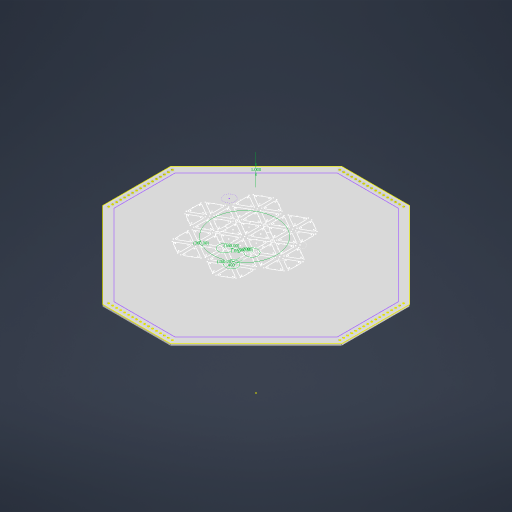
# Autodesk Inventor part: Belly Pan
Saved by Autodesk Inventor 2024.3 (Build 283343000, 343)
## iProperties
Created: 2024-11-27
Part Number: Belly Pan
Material: Generic
Document SubType Name: Modeling
Designer: kaito
Density: 1 g/cm^3
Appearance: Default
Author: kaito
Autodesk Inventor part; units mm, degrees
(part 1 of 2)
ref_plane "YZ Plane" through (0, 0, 0) normal (1, 0, 0) x (0, 1, 0)
ref_plane "XZ Plane" through (0, 0, 0) normal (0, 1, 0) x (-1, 0, 0)
ref_plane "XY Plane" through (0, 0, 0) normal (0, 0, 1) x (1, 0, 0)
sketch "Sketch1" plane through (0, 0, 0) normal (0, 1, 0) x (-1, 0, 0)
  line L0 (0, 0) -> (762, 0) construction
  line L1 (762, 0) -> (762, -762)
  line L2 (762, -762) -> (0, -762)
  line L3 (762, -273.05) -> (736.6, -273.05) construction
  line L4 (736.6, -273.05) -> (736.6, -488.95) construction
  line L5 (736.6, -488.95) -> (762, -488.95) construction
  line L6 (762, -488.95) -> (762, -273.05) construction
  line L7 (488.95, 0) -> (273.05, 0)
  line L8 (273.05, 0) -> (273.05, -25.4) construction
  line L9 (273.05, -25.4) -> (488.95, -25.4) construction
  line L10 (488.95, -25.4) -> (488.95, 0) construction
  line L11 (488.95, -762) -> (273.05, -762) construction
  line L12 (273.05, -762) -> (273.05, -736.6) construction
  line L13 (273.05, -736.6) -> (488.95, -736.6) construction
  line L14 (488.95, -736.6) -> (488.95, -762) construction
  line L15 (0, 0) -> (0, -762)
  line L16 (0, -273.05) -> (25.4, -273.05) construction
  line L17 (25.4, -273.05) -> (25.4, -488.95) construction
  line L18 (25.4, -488.95) -> (0, -488.95) construction
  line L19 (0, -488.95) -> (0, -273.05) construction
  line L20 (273.05, 0) -> (0, -273.05)
  line L21 (488.95, 0) -> (762, -273.05)
  line L22 (762, -488.95) -> (488.95, -762)
  line L23 (0, -488.95) -> (273.05, -762)
  circle A0 centre (482.6, -12.7) radius 2.4892
  circle A1 centre (469.9, -12.7) radius 2.4892
  circle A2 centre (457.2, -12.7) radius 2.4892
  circle A3 centre (444.5, -12.7) radius 2.4892
  circle A4 centre (431.8, -12.7) radius 2.4892
  circle A5 centre (419.1, -12.7) radius 2.4892
  circle A6 centre (406.4, -12.7) radius 2.4892
  circle A7 centre (393.7, -12.7) radius 2.4892
  circle A8 centre (381, -12.7) radius 2.4892
  circle A9 centre (368.3, -12.7) radius 2.4892
  circle A10 centre (355.6, -12.7) radius 2.4892
  circle A11 centre (342.9, -12.7) radius 2.4892
  circle A12 centre (330.2, -12.7) radius 2.4892
  circle A13 centre (317.5, -12.7) radius 2.4892
  circle A14 centre (304.8, -12.7) radius 2.4892
  circle A15 centre (292.1, -12.7) radius 2.4892
  circle A16 centre (279.4, -12.7) radius 2.4892
  circle A17 centre (749.3, -279.4) radius 2.4892
  circle A18 centre (749.3, -292.1) radius 2.4892
  circle A19 centre (749.3, -304.8) radius 2.4892
  circle A20 centre (749.3, -317.5) radius 2.4892
  circle A21 centre (749.3, -330.2) radius 2.4892
  circle A22 centre (749.3, -342.9) radius 2.4892
  circle A23 centre (749.3, -355.6) radius 2.4892
  circle A24 centre (749.3, -368.3) radius 2.4892
  circle A25 centre (749.3, -381) radius 2.4892
  circle A26 centre (749.3, -393.7) radius 2.4892
  circle A27 centre (749.3, -406.4) radius 2.4892
  circle A28 centre (749.3, -419.1) radius 2.4892
  circle A29 centre (749.3, -431.8) radius 2.4892
  circle A30 centre (749.3, -444.5) radius 2.4892
  circle A31 centre (749.3, -457.2) radius 2.4892
  circle A32 centre (749.3, -469.9) radius 2.4892
  circle A33 centre (749.3, -482.6) radius 2.4892
  circle A34 centre (482.6, -749.3) radius 2.4892
  circle A35 centre (469.9, -749.3) radius 2.4892
  circle A36 centre (457.2, -749.3) radius 2.4892
  circle A37 centre (444.5, -749.3) radius 2.4892
  circle A38 centre (431.8, -749.3) radius 2.4892
  circle A39 centre (419.1, -749.3) radius 2.4892
  circle A40 centre (406.4, -749.3) radius 2.4892
  circle A41 centre (393.7, -749.3) radius 2.4892
  circle A42 centre (381, -749.3) radius 2.4892
  circle A43 centre (368.3, -749.3) radius 2.4892
  circle A44 centre (355.6, -749.3) radius 2.4892
  circle A45 centre (342.9, -749.3) radius 2.4892
  circle A46 centre (330.2, -749.3) radius 2.4892
  circle A47 centre (317.5, -749.3) radius 2.4892
  circle A48 centre (304.8, -749.3) radius 2.4892
  circle A49 centre (292.1, -749.3) radius 2.4892
  circle A50 centre (279.4, -749.3) radius 2.4892
  circle A51 centre (12.7, -279.4) radius 2.4892
  circle A52 centre (12.7, -292.1) radius 2.4892
  circle A53 centre (12.7, -304.8) radius 2.4892
  circle A54 centre (12.7, -317.5) radius 2.4892
  circle A55 centre (12.7, -330.2) radius 2.4892
  circle A56 centre (12.7, -342.9) radius 2.4892
  circle A57 centre (12.7, -355.6) radius 2.4892
  circle A58 centre (12.7, -368.3) radius 2.4892
  circle A59 centre (12.7, -381) radius 2.4892
  circle A60 centre (12.7, -393.7) radius 2.4892
  circle A61 centre (12.7, -406.4) radius 2.4892
  circle A62 centre (12.7, -419.1) radius 2.4892
  circle A63 centre (12.7, -431.8) radius 2.4892
  circle A64 centre (12.7, -444.5) radius 2.4892
  circle A65 centre (12.7, -457.2) radius 2.4892
  circle A66 centre (12.7, -469.9) radius 2.4892
  circle A67 centre (12.7, -482.6) radius 2.4892
  point P0 (736.6, -381)
  point P1 (381, -25.4)
  point P2 (381, 0)
  point P3 (381, -736.6)
  point P4 (381, -762)
  point P5 (25.4, -381)
  point P6 (0, -381)
  point P7 (762, -381)
  point P8 (12.7, -273.05)
  point P9 (12.7, -488.95)
  point P10 (488.95, -12.7)
  point P11 (749.3, -273.05)
  point P12 (488.95, -749.3)
  point P13 (273.05, -762)
  point P14 (762, -488.95)
  point P15 (0, -381)
  dimension "d0" = 762
  dimension "d1" = 762
  dimension "d4" = 25.4
  dimension "d5" = 215.9
  dimension "d6" = 25.4
  dimension "d7" = 215.9
  dimension "d8" = 25.4
  dimension "d9" = 25.4
  dimension "d11" = 215.9
  dimension "d22" = 4.9784
  dimension "d23" = 6.35
  dimension "d26" = 12.7
  dimension "d31" = 4.9784
  dimension "d32" = 6.35
  dimension "d35" = 12.7
  dimension "d40" = 4.9784
  dimension "d41" = 6.35
  dimension "d44" = 12.7
  dimension "d51" = 215.9
  dimension "d60" = 4.9784
  dimension "d63" = 12.7
  constraints: 68 centre point, 48 end point, 14 midpoint, 9 parallel, 7 horizontal, 5 horizontal alignment, 5 perpendicular, 4 point on line, 4 vertical alignment, 3 vertical, 128 other
  measures "d0" distance of L1.end L2.end
  measures "d1" distance of L0.end L1.end
  measures "d4" distance of L5.end L4.end
  measures "d5" distance of L9.end L8.end
  measures "d6" distance of L8.end L7.end
  measures "d7" distance of L12.end L13.end
  measures "d8" distance of L11.end L12.end
  measures "d9" distance of L17.end L18.end
  measures "d11" distance of L3.end L4.end
  measures "d22" diameter of A0
  measures "d23" distance from line of L10 A0.centre
  measures "d26" distance of A0.centre A1.centre
  measures "d31" diameter of A17
  measures "d32" distance of point (749.3, -273.05) A17.centre
  measures "d35" distance of A17.centre A18.centre
  measures "d40" diameter of A34
  measures "d41" distance of A34.centre point (488.95, -749.3)
  measures "d44" distance of A34.centre A35.centre
  measures "d51" distance of L16.end L17.end
  measures "d60" diameter of A51
  measures "d63" distance of A51.centre A52.centre
extrude "Extrusion1" add sketch "Sketch1" along normal blind 6.35 contours L1 L22 L2 L23 L15 L20 L7 L21
sketch "Sketch3" plane through (0, 6.35, 0) normal (0, 1, 0) x (1, 0, 0)
  line L0 (-762, 488.95) -> (-762, 273.05) projected
  line L1 (-762, 273.05) -> (-488.95, 0) projected
  line L2 (-273.05, 0) -> (0, 273.05) projected
  line L3 (0, 273.05) -> (0, 488.95) projected
  line L4 (0, 488.95) -> (-273.05, 762) projected
  line L5 (-273.05, 762) -> (-488.95, 762) projected
  line L6 (-488.95, 762) -> (-762, 488.95) projected
  line L7 (-762, 488.95) -> (-762, 273.05) projected
  line L8 (-762, 273.05) -> (-488.95, 0) projected
  line L9 (-488.95, 0) -> (-273.05, 0) projected
  circle A0 centre (-12.7, 482.6) radius 2.4892 projected
  circle A1 centre (-12.7, 457.2) radius 2.4892 projected
  circle A2 centre (-12.7, 431.8) radius 2.4892 projected
  circle A3 centre (-12.7, 406.4) radius 2.4892 projected
  circle A4 centre (-12.7, 381) radius 2.4892 projected
  circle A5 centre (-12.7, 355.6) radius 2.4892 projected
  circle A6 centre (-12.7, 330.2) radius 2.4892 projected
  circle A7 centre (-12.7, 304.8) radius 2.4892 projected
  circle A8 centre (-12.7, 279.4) radius 2.4892 projected
  circle A9 centre (-292.1, 749.3) radius 2.4892 projected
  circle A10 centre (-317.5, 749.3) radius 2.4892 projected
  circle A11 centre (-342.9, 749.3) radius 2.4892 projected
  circle A12 centre (-368.3, 749.3) radius 2.4892 projected
  circle A13 centre (-393.7, 749.3) radius 2.4892 projected
  circle A14 centre (-419.1, 749.3) radius 2.4892 projected
  circle A15 centre (-444.5, 749.3) radius 2.4892 projected
  circle A16 centre (-469.9, 749.3) radius 2.4892 projected
  circle A17 centre (-749.3, 482.6) radius 2.4892 projected
  circle A18 centre (-749.3, 457.2) radius 2.4892 projected
  circle A19 centre (-749.3, 431.8) radius 2.4892 projected
  circle A20 centre (-749.3, 406.4) radius 2.4892 projected
  circle A21 centre (-749.3, 381) radius 2.4892 projected
  circle A22 centre (-749.3, 355.6) radius 2.4892 projected
  circle A23 centre (-749.3, 330.2) radius 2.4892 projected
  circle A24 centre (-749.3, 304.8) radius 2.4892 projected
  circle A25 centre (-749.3, 279.4) radius 2.4892 projected
  circle A26 centre (-292.1, 12.7) radius 2.4892 projected
  circle A27 centre (-317.5, 12.7) radius 2.4892 projected
  circle A28 centre (-342.9, 12.7) radius 2.4892 projected
  circle A29 centre (-368.3, 12.7) radius 2.4892 projected
  circle A30 centre (-393.7, 12.7) radius 2.4892 projected
  circle A31 centre (-482.6, 12.7) radius 2.4892 projected
  circle A32 centre (-469.9, 12.7) radius 2.4892 projected
  circle A33 centre (-457.2, 12.7) radius 2.4892 projected
  circle A34 centre (-444.5, 12.7) radius 2.4892 projected
  circle A35 centre (-431.8, 12.7) radius 2.4892 projected
  circle A36 centre (-419.1, 12.7) radius 2.4892 projected
  circle A37 centre (-406.4, 12.7) radius 2.4892 projected
  circle A38 centre (-381, 12.7) radius 2.4892 projected
  circle A39 centre (-355.6, 12.7) radius 2.4892 projected
  circle A40 centre (-330.2, 12.7) radius 2.4892 projected
  circle A41 centre (-304.8, 12.7) radius 2.4892 projected
  circle A42 centre (-279.4, 12.7) radius 2.4892 projected
  circle A43 centre (-749.3, 292.1) radius 2.4892 projected
  circle A44 centre (-749.3, 317.5) radius 2.4892 projected
  circle A45 centre (-749.3, 342.9) radius 2.4892 projected
  circle A46 centre (-749.3, 368.3) radius 2.4892 projected
  circle A47 centre (-749.3, 393.7) radius 2.4892 projected
  circle A48 centre (-749.3, 419.1) radius 2.4892 projected
  circle A49 centre (-749.3, 444.5) radius 2.4892 projected
  circle A50 centre (-749.3, 469.9) radius 2.4892 projected
  circle A51 centre (-482.6, 749.3) radius 2.4892 projected
  circle A52 centre (-457.2, 749.3) radius 2.4892 projected
  circle A53 centre (-431.8, 749.3) radius 2.4892 projected
  circle A54 centre (-406.4, 749.3) radius 2.4892 projected
  circle A55 centre (-381, 749.3) radius 2.4892 projected
  circle A56 centre (-355.6, 749.3) radius 2.4892 projected
  circle A57 centre (-330.2, 749.3) radius 2.4892 projected
  circle A58 centre (-304.8, 749.3) radius 2.4892 projected
  circle A59 centre (-279.4, 749.3) radius 2.4892 projected
  circle A60 centre (-12.7, 292.1) radius 2.4892 projected
  circle A61 centre (-12.7, 317.5) radius 2.4892 projected
  circle A62 centre (-12.7, 342.9) radius 2.4892 projected
  circle A63 centre (-12.7, 368.3) radius 2.4892 projected
  circle A64 centre (-12.7, 393.7) radius 2.4892 projected
  circle A65 centre (-12.7, 419.1) radius 2.4892 projected
  circle A66 centre (-12.7, 444.5) radius 2.4892 projected
  circle A67 centre (-12.7, 469.9) radius 2.4892 projected
  line L10 (-736.6, 478.429) -> (-478.429, 736.6)
  line L11 (-478.429, 736.6) -> (-283.571, 736.6)
  line L12 (-283.571, 736.6) -> (-25.4, 478.429)
  line L13 (-25.4, 478.429) -> (-25.4, 283.571)
  line L14 (-25.4, 283.571) -> (-283.571, 25.4)
  line L15 (-283.571, 25.4) -> (-478.429, 25.4)
  line L16 (-478.429, 25.4) -> (-736.6, 283.571)
  line L17 (-736.6, 283.571) -> (-736.6, 478.429)
  circle A68 centre (-393.7, 381) radius 15.24 construction
  line L18 (-411.48, 376.6006) -> (-436.88, 361.9359)
  line L19 (-444.5, 366.3353) -> (-444.5, 395.6647)
  line L20 (-436.88, 400.0641) -> (-411.48, 385.3994)
  arc A69 (-411.48, 376.6006) -> (-411.48, 385.3994) centre (-414.02, 381) ccw
  arc A70 (-444.5, 366.3353) -> (-436.88, 361.9359) centre (-439.42, 366.3353) ccw
  arc A71 (-436.88, 400.0641) -> (-444.5, 395.6647) centre (-439.42, 395.6647) ccw
  line L21 (-398.78, 363.4024) -> (-398.78, 334.073)
  arc A72 (-406.4, 329.6736) -> (-398.78, 334.073) centre (-403.86, 334.073) ccw
  line L22 (-406.4, 329.6736) -> (-431.8, 344.3383)
  arc A73 (-431.8, 353.1371) -> (-431.8, 344.3383) centre (-429.26, 348.7377) ccw
  line L23 (-431.8, 353.1371) -> (-406.4, 367.8018)
  arc A74 (-398.78, 363.4024) -> (-406.4, 367.8018) centre (-403.86, 363.4024) ccw
  line L24 (-381, 367.8018) -> (-355.6, 353.1371)
  arc A75 (-355.6, 344.3383) -> (-355.6, 353.1371) centre (-358.14, 348.7377) ccw
  line L25 (-355.6, 344.3383) -> (-381, 329.6736)
  arc A76 (-388.62, 334.073) -> (-381, 329.6736) centre (-383.54, 334.073) ccw
  line L26 (-388.62, 334.073) -> (-388.62, 363.4024)
  arc A77 (-381, 367.8018) -> (-388.62, 363.4024) centre (-383.54, 363.4024) ccw
  line L27 (-375.92, 385.3994) -> (-350.52, 400.0641)
  arc A78 (-342.9, 395.6647) -> (-350.52, 400.0641) centre (-347.98, 395.6647) ccw
  line L28 (-342.9, 395.6647) -> (-342.9, 366.3353)
  arc A79 (-350.52, 361.9359) -> (-342.9, 366.3353) centre (-347.98, 366.3353) ccw
  line L29 (-350.52, 361.9359) -> (-375.92, 376.6006)
  arc A80 (-375.92, 385.3994) -> (-375.92, 376.6006) centre (-373.38, 381) ccw
  line L30 (-388.62, 398.5976) -> (-388.62, 427.927)
  arc A81 (-381, 432.3264) -> (-388.62, 427.927) centre (-383.54, 427.927) ccw
  line L31 (-381, 432.3264) -> (-355.6, 417.6617)
  arc A82 (-355.6, 408.8629) -> (-355.6, 417.6617) centre (-358.14, 413.2623) ccw
  line L32 (-355.6, 408.8629) -> (-381, 394.1982)
  arc A83 (-388.62, 398.5976) -> (-381, 394.1982) centre (-383.54, 398.5976) ccw
  line L33 (-406.4, 394.1982) -> (-431.8, 408.8629)
  arc A84 (-431.8, 417.6617) -> (-431.8, 408.8629) centre (-429.26, 413.2623) ccw
  line L34 (-431.8, 417.6617) -> (-406.4, 432.3264)
  arc A85 (-398.78, 427.927) -> (-406.4, 432.3264) centre (-403.86, 427.927) ccw
  line L35 (-398.78, 427.927) -> (-398.78, 398.5976)
  arc A86 (-406.4, 394.1982) -> (-398.78, 398.5976) centre (-403.86, 398.5976) ccw
  line L36 (-416.56, 361.9359) -> (-421.64, 370.7347)
  circle A87 centre (-393.7, 381) radius 5.08
  line L37 (-408.94, 381) -> (-398.78, 381)
  circle A88 centre (-449.58, 348.7377) radius 15.24 construction
  line L38 (-462.28, 361.9359) -> (-487.68, 376.6006)
  arc A89 (-462.28, 361.9359) -> (-454.66, 366.3353) centre (-459.74, 366.3353) ccw
  line L39 (-454.66, 395.6647) -> (-454.66, 366.3353)
  arc A90 (-454.66, 395.6647) -> (-462.28, 400.0641) centre (-459.74, 395.6647) ccw
  line L40 (-487.68, 385.3994) -> (-462.28, 400.0641)
  arc A91 (-487.68, 385.3994) -> (-487.68, 376.6006) centre (-485.14, 381) ccw
  line L41 (-467.36, 344.3383) -> (-492.76, 329.6736)
  arc A92 (-467.36, 344.3383) -> (-467.36, 353.1371) centre (-469.9, 348.7377) ccw
  line L42 (-492.76, 367.8018) -> (-467.36, 353.1371)
  arc A93 (-492.76, 367.8018) -> (-500.38, 363.4024) centre (-495.3, 363.4024) ccw
  line L43 (-500.38, 334.073) -> (-500.38, 363.4024)
  arc A94 (-500.38, 334.073) -> (-492.76, 329.6736) centre (-495.3, 334.073) ccw
  line L44 (-454.66, 331.14) -> (-454.66, 301.8106)
  arc A95 (-454.66, 331.14) -> (-462.28, 335.5394) centre (-459.74, 331.14) ccw
  line L45 (-487.68, 320.8747) -> (-462.28, 335.5394)
  arc A96 (-487.68, 320.8747) -> (-487.68, 312.0759) centre (-485.14, 316.4753) ccw
  line L46 (-462.28, 297.4112) -> (-487.68, 312.0759)
  arc A97 (-462.28, 297.4112) -> (-454.66, 301.8106) centre (-459.74, 301.8106) ccw
  line L47 (-436.88, 335.5394) -> (-411.48, 320.8747)
  arc A98 (-436.88, 335.5394) -> (-444.5, 331.14) centre (-439.42, 331.14) ccw
  line L48 (-444.5, 301.8106) -> (-444.5, 331.14)
  arc A99 (-444.5, 301.8106) -> (-436.88, 297.4112) centre (-439.42, 301.8106) ccw
  line L49 (-411.48, 312.0759) -> (-436.88, 297.4112)
  arc A100 (-411.48, 312.0759) -> (-411.48, 320.8747) centre (-414.02, 316.4753) ccw
  line L50 (-431.8, 353.1371) -> (-406.4, 367.8018)
  arc A101 (-431.8, 353.1371) -> (-431.8, 344.3383) centre (-429.26, 348.7377) ccw
  line L51 (-406.4, 329.6736) -> (-431.8, 344.3383)
  arc A102 (-406.4, 329.6736) -> (-398.78, 334.073) centre (-403.86, 334.073) ccw
  line L52 (-398.78, 363.4024) -> (-398.78, 334.073)
  arc A103 (-398.78, 363.4024) -> (-406.4, 367.8018) centre (-403.86, 363.4024) ccw
  circle A104 centre (-393.7, 316.4753) radius 15.24 construction
  line L53 (-398.78, 298.8777) -> (-398.78, 269.5483)
  line L54 (-406.4, 265.1489) -> (-431.8, 279.8136)
  arc A105 (-406.4, 265.1489) -> (-398.78, 269.5483) centre (-403.86, 269.5483) ccw
  line L55 (-431.8, 288.6124) -> (-406.4, 303.2771)
  arc A106 (-398.78, 298.8777) -> (-406.4, 303.2771) centre (-403.86, 298.8777) ccw
  arc A107 (-431.8, 288.6124) -> (-431.8, 279.8136) centre (-429.26, 284.213) ccw
  line L56 (-381, 303.2771) -> (-355.6, 288.6124)
  line L57 (-355.6, 279.8136) -> (-381, 265.1489)
  arc A108 (-355.6, 279.8136) -> (-355.6, 288.6124) centre (-358.14, 284.213) ccw
  line L58 (-388.62, 269.5483) -> (-388.62, 298.8777)
  arc A109 (-381, 303.2771) -> (-388.62, 298.8777) centre (-383.54, 298.8777) ccw
  arc A110 (-388.62, 269.5483) -> (-381, 265.1489) centre (-383.54, 269.5483) ccw
  line L59 (-375.92, 320.8747) -> (-350.52, 335.5394)
  line L60 (-342.9, 331.14) -> (-342.9, 301.8106)
  arc A111 (-342.9, 331.14) -> (-350.52, 335.5394) centre (-347.98, 331.14) ccw
  line L61 (-350.52, 297.4112) -> (-375.92, 312.0759)
  arc A112 (-375.92, 320.8747) -> (-375.92, 312.0759) centre (-373.38, 316.4753) ccw
  arc A113 (-350.52, 297.4112) -> (-342.9, 301.8106) centre (-347.98, 301.8106) ccw
  line L62 (-388.62, 334.073) -> (-388.62, 363.4024)
  line L63 (-381, 367.8018) -> (-355.6, 353.1371)
  arc A114 (-381, 367.8018) -> (-388.62, 363.4024) centre (-383.54, 363.4024) ccw
  line L64 (-355.6, 344.3383) -> (-381, 329.6736)
  arc A115 (-388.62, 334.073) -> (-381, 329.6736) centre (-383.54, 334.073) ccw
  arc A116 (-355.6, 344.3383) -> (-355.6, 353.1371) centre (-358.14, 348.7377) ccw
  line L65 (-406.4, 329.6736) -> (-431.8, 344.3383)
  line L66 (-431.8, 353.1371) -> (-406.4, 367.8018)
  arc A117 (-431.8, 353.1371) -> (-431.8, 344.3383) centre (-429.26, 348.7377) ccw
  line L67 (-398.78, 363.4024) -> (-398.78, 334.073)
  arc A118 (-406.4, 329.6736) -> (-398.78, 334.073) centre (-403.86, 334.073) ccw
  arc A119 (-398.78, 363.4024) -> (-406.4, 367.8018) centre (-403.86, 363.4024) ccw
  circle A120 centre (-449.58, 413.2623) radius 15.24 construction
  arc A121 (-406.4, 329.6736) -> (-398.78, 334.073) centre (-403.86, 334.073) ccw
  line L68 (-406.4, 329.6736) -> (-431.8, 344.3383)
  arc A122 (-431.8, 353.1371) -> (-431.8, 344.3383) centre (-429.26, 348.7377) ccw
  arc A123 (-299.72, 376.6006) -> (-299.72, 385.3994) centre (-302.26, 381) ccw
  arc A124 (-444.5, 366.3353) -> (-436.88, 361.9359) centre (-439.42, 366.3353) ccw
  line L69 (-398.78, 363.4024) -> (-398.78, 334.073)
  line L70 (-431.8, 353.1371) -> (-406.4, 367.8018)
  arc A125 (-398.78, 363.4024) -> (-406.4, 367.8018) centre (-403.86, 363.4024) ccw
  line L71 (-411.48, 376.6006) -> (-436.88, 361.9359)
  line L72 (-444.5, 366.3353) -> (-444.5, 395.6647)
  line L73 (-431.8, 482.1864) -> (-406.4, 496.8511)
  arc A126 (-398.78, 492.4517) -> (-406.4, 496.8511) centre (-403.86, 492.4517) ccw
  line L74 (-406.4, 458.7229) -> (-431.8, 473.3876)
  line L75 (-398.78, 492.4517) -> (-398.78, 463.1223)
  arc A127 (-406.4, 458.7229) -> (-398.78, 463.1223) centre (-403.86, 463.1223) ccw
  line L76 (-388.62, 463.1223) -> (-388.62, 492.4517)
  arc A128 (-388.62, 463.1223) -> (-381, 458.7229) centre (-383.54, 463.1223) ccw
  line L77 (-381, 496.8511) -> (-355.6, 482.1864)
  arc A129 (-381, 496.8511) -> (-388.62, 492.4517) centre (-383.54, 492.4517) ccw
  circle A130 centre (-393.7, 445.5247) radius 15.24 construction
  line L78 (-401.32, 432.3264) -> (-396.24, 441.1253)
  arc A131 (-398.78, 427.927) -> (-406.4, 432.3264) centre (-403.86, 427.927) ccw
  circle A132 centre (-393.7, 445.5247) radius 5.08
  line L79 (-375.92, 449.9241) -> (-350.52, 464.5888)
  arc A133 (-342.9, 460.1894) -> (-350.52, 464.5888) centre (-347.98, 460.1894) ccw
  line L80 (-342.9, 460.1894) -> (-342.9, 430.86)
  line L81 (-342.9, 460.1894) -> (-342.9, 430.86)
  arc A134 (-375.92, 449.9241) -> (-375.92, 441.1253) centre (-373.38, 445.5247) ccw
  arc A135 (-375.92, 449.9241) -> (-375.92, 441.1253) centre (-373.38, 445.5247) ccw
  line L82 (-375.92, 449.9241) -> (-350.52, 464.5888)
  arc A136 (-355.6, 473.3876) -> (-355.6, 482.1864) centre (-358.14, 477.787) ccw
  line L83 (-355.6, 473.3876) -> (-381, 458.7229)
  arc A137 (-355.6, 408.8629) -> (-355.6, 417.6617) centre (-358.14, 413.2623) ccw
  arc A138 (-320.04, 417.6617) -> (-320.04, 408.8629) centre (-317.5, 413.2623) ccw
  arc A139 (-350.52, 426.4606) -> (-342.9, 430.86) centre (-347.98, 430.86) ccw
  circle A140 centre (-337.82, 413.2623) radius 15.24 construction
  arc A141 (-342.9, 395.6647) -> (-350.52, 400.0641) centre (-347.98, 395.6647) ccw
  arc A142 (-355.6, 408.8629) -> (-355.6, 417.6617) centre (-358.14, 413.2623) ccw
  arc A143 (-381, 432.3264) -> (-388.62, 427.927) centre (-383.54, 427.927) ccw
  arc A144 (-381, 432.3264) -> (-388.62, 427.927) centre (-383.54, 427.927) ccw
  arc A145 (-381, 432.3264) -> (-388.62, 427.927) centre (-383.54, 427.927) ccw
  arc A146 (-431.8, 482.1864) -> (-431.8, 473.3876) centre (-429.26, 477.787) ccw
  line L84 (-406.4, 394.1982) -> (-431.8, 408.8629)
  arc A147 (-406.4, 394.1982) -> (-398.78, 398.5976) centre (-403.86, 398.5976) ccw
  arc A148 (-431.8, 417.6617) -> (-431.8, 408.8629) centre (-429.26, 413.2623) ccw
  arc A149 (-411.48, 376.6006) -> (-411.48, 385.3994) centre (-414.02, 381) ccw
  line L85 (-436.88, 400.0641) -> (-411.48, 385.3994)
  arc A150 (-436.88, 400.0641) -> (-444.5, 395.6647) centre (-439.42, 395.6647) ccw
  arc A151 (-444.5, 430.86) -> (-436.88, 426.4606) centre (-439.42, 430.86) ccw
  circle A152 centre (-449.58, 413.2623) radius 15.24 construction
  line L86 (-431.8, 417.6617) -> (-406.4, 432.3264)
  arc A153 (-411.48, 441.1253) -> (-411.48, 449.9241) centre (-414.02, 445.5247) ccw
  line L87 (-411.48, 441.1253) -> (-436.88, 426.4606)
  line L88 (-436.88, 464.5888) -> (-411.48, 449.9241)
  line L89 (-444.5, 430.86) -> (-444.5, 460.1894)
  arc A154 (-436.88, 464.5888) -> (-444.5, 460.1894) centre (-439.42, 460.1894) ccw
  circle A155 centre (-393.7, 381) radius 15.24 construction
  arc A156 (-381, 367.8018) -> (-388.62, 363.4024) centre (-383.54, 363.4024) ccw
  arc A157 (-375.92, 385.3994) -> (-375.92, 376.6006) centre (-373.38, 381) ccw
  arc A158 (-388.62, 334.073) -> (-381, 329.6736) centre (-383.54, 334.073) ccw
  line L90 (-388.62, 334.073) -> (-388.62, 363.4024)
  line L91 (-355.6, 344.3383) -> (-381, 329.6736)
  line L92 (-381, 367.8018) -> (-355.6, 353.1371)
  line L93 (-350.52, 361.9359) -> (-375.92, 376.6006)
  arc A159 (-355.6, 344.3383) -> (-355.6, 353.1371) centre (-358.14, 348.7377) ccw
  arc A160 (-350.52, 361.9359) -> (-342.9, 366.3353) centre (-347.98, 366.3353) ccw
  line L94 (-375.92, 385.3994) -> (-350.52, 400.0641)
  line L95 (-342.9, 395.6647) -> (-342.9, 366.3353)
  arc A161 (-332.74, 366.3353) -> (-325.12, 361.9359) centre (-327.66, 366.3353) ccw
  line L96 (-332.74, 366.3353) -> (-332.74, 395.6647)
  arc A162 (-325.12, 400.0641) -> (-332.74, 395.6647) centre (-327.66, 395.6647) ccw
  line L97 (-299.72, 376.6006) -> (-325.12, 361.9359)
  line L98 (-325.12, 400.0641) -> (-299.72, 385.3994)
  line L99 (-294.64, 394.1982) -> (-320.04, 408.8629)
  arc A163 (-294.64, 394.1982) -> (-287.02, 398.5976) centre (-292.1, 398.5976) ccw
  line L100 (-287.02, 427.927) -> (-287.02, 398.5976)
  arc A164 (-287.02, 427.927) -> (-294.64, 432.3264) centre (-292.1, 427.927) ccw
  line L101 (-320.04, 417.6617) -> (-294.64, 432.3264)
  arc A165 (-325.12, 464.5888) -> (-332.74, 460.1894) centre (-327.66, 460.1894) ccw
  arc A166 (-342.9, 460.1894) -> (-350.52, 464.5888) centre (-347.98, 460.1894) ccw
  arc A167 (-332.74, 430.86) -> (-325.12, 426.4606) centre (-327.66, 430.86) ccw
  line L102 (-332.74, 430.86) -> (-332.74, 460.1894)
  line L103 (-299.72, 441.1253) -> (-325.12, 426.4606)
  line L104 (-325.12, 464.5888) -> (-299.72, 449.9241)
  arc A168 (-299.72, 441.1253) -> (-299.72, 449.9241) centre (-302.26, 445.5247) ccw
  line L105 (-398.78, 427.927) -> (-398.78, 398.5976)
  line L106 (-355.6, 408.8629) -> (-381, 394.1982)
  arc A169 (-388.62, 398.5976) -> (-381, 394.1982) centre (-383.54, 398.5976) ccw
  line L107 (-388.62, 398.5976) -> (-388.62, 427.927)
  line L108 (-388.62, 416.1953) -> (-398.78, 416.1953)
  arc A170 (-388.62, 398.5976) -> (-381, 394.1982) centre (-383.54, 398.5976) ccw
  arc A171 (-388.62, 398.5976) -> (-381, 394.1982) centre (-383.54, 398.5976) ccw
  line L109 (-388.62, 398.5976) -> (-388.62, 427.927)
  line L110 (-388.62, 398.5976) -> (-388.62, 427.927)
  line L111 (-355.6, 408.8629) -> (-381, 394.1982)
  line L112 (-355.6, 408.8629) -> (-381, 394.1982)
  line L113 (-381, 432.3264) -> (-355.6, 417.6617)
  line L114 (-350.52, 426.4606) -> (-375.92, 441.1253)
  line L115 (-350.52, 426.4606) -> (-375.92, 441.1253)
  line L116 (-381, 432.3264) -> (-355.6, 417.6617)
  line L117 (-381, 432.3264) -> (-355.6, 417.6617)
  arc A172 (-350.52, 426.4606) -> (-342.9, 430.86) centre (-347.98, 430.86) ccw
  arc A173 (-355.6, 408.8629) -> (-355.6, 417.6617) centre (-358.14, 413.2623) ccw
  arc A174 (-355.6, 408.8629) -> (-355.6, 417.6617) centre (-358.14, 413.2623) ccw
  line L118 (-355.6, 408.8629) -> (-381, 394.1982)
  arc A175 (-388.62, 398.5976) -> (-381, 394.1982) centre (-383.54, 398.5976) ccw
  arc A176 (-342.9, 524.714) -> (-350.52, 529.1134) centre (-347.98, 524.714) ccw
  arc A177 (-406.4, 394.1982) -> (-398.78, 398.5976) centre (-403.86, 398.5976) ccw
  line L119 (-381, 432.3264) -> (-355.6, 417.6617)
  line L120 (-388.62, 398.5976) -> (-388.62, 427.927)
  arc A178 (-381, 432.3264) -> (-388.62, 427.927) centre (-383.54, 427.927) ccw
  line L121 (-398.78, 427.927) -> (-398.78, 398.5976)
  line L122 (-406.4, 394.1982) -> (-431.8, 408.8629)
  line L123 (-500.38, 463.1223) -> (-500.38, 492.4517)
  arc A179 (-492.76, 496.8511) -> (-500.38, 492.4517) centre (-495.3, 492.4517) ccw
  line L124 (-467.36, 473.3876) -> (-492.76, 458.7229)
  line L125 (-492.76, 496.8511) -> (-467.36, 482.1864)
  arc A180 (-467.36, 473.3876) -> (-467.36, 482.1864) centre (-469.9, 477.787) ccw
  line L126 (-462.28, 490.9852) -> (-487.68, 505.6499)
  arc A181 (-462.28, 490.9852) -> (-454.66, 495.3846) centre (-459.74, 495.3846) ccw
  line L127 (-487.68, 514.4487) -> (-462.28, 529.1134)
  arc A182 (-487.68, 514.4487) -> (-487.68, 505.6499) centre (-485.14, 510.0493) ccw
  circle A183 centre (-449.58, 477.787) radius 15.24 construction
  line L128 (-441.96, 464.5888) -> (-447.04, 473.3876)
  arc A184 (-436.88, 464.5888) -> (-444.5, 460.1894) centre (-439.42, 460.1894) ccw
  circle A185 centre (-449.58, 477.787) radius 5.08
  line L129 (-444.5, 495.3846) -> (-444.5, 524.714)
  arc A186 (-436.88, 529.1134) -> (-444.5, 524.714) centre (-439.42, 524.714) ccw
  line L130 (-436.88, 529.1134) -> (-411.48, 514.4487)
  line L131 (-436.88, 529.1134) -> (-411.48, 514.4487)
  arc A187 (-444.5, 495.3846) -> (-436.88, 490.9852) centre (-439.42, 495.3846) ccw
  arc A188 (-444.5, 495.3846) -> (-436.88, 490.9852) centre (-439.42, 495.3846) ccw
  line L132 (-444.5, 495.3846) -> (-444.5, 524.714)
  arc A189 (-454.66, 524.714) -> (-462.28, 529.1134) centre (-459.74, 524.714) ccw
  line L133 (-454.66, 524.714) -> (-454.66, 495.3846)
  arc A190 (-398.78, 492.4517) -> (-406.4, 496.8511) centre (-403.86, 492.4517) ccw
  arc A191 (-388.62, 527.647) -> (-381, 523.2476) centre (-383.54, 527.647) ccw
  arc A192 (-411.48, 505.6499) -> (-411.48, 514.4487) centre (-414.02, 510.0493) ccw
  circle A193 centre (-393.7, 510.0493) radius 15.24 construction
  arc A194 (-381, 496.8511) -> (-388.62, 492.4517) centre (-383.54, 492.4517) ccw
  arc A195 (-398.78, 492.4517) -> (-406.4, 496.8511) centre (-403.86, 492.4517) ccw
  arc A196 (-431.8, 482.1864) -> (-431.8, 473.3876) centre (-429.26, 477.787) ccw
  arc A197 (-431.8, 482.1864) -> (-431.8, 473.3876) centre (-429.26, 477.787) ccw
  arc A198 (-431.8, 482.1864) -> (-431.8, 473.3876) centre (-429.26, 477.787) ccw
  arc A199 (-500.38, 463.1223) -> (-492.76, 458.7229) centre (-495.3, 463.1223) ccw
  line L134 (-411.48, 441.1253) -> (-436.88, 426.4606)
  arc A200 (-411.48, 441.1253) -> (-411.48, 449.9241) centre (-414.02, 445.5247) ccw
  arc A201 (-444.5, 430.86) -> (-436.88, 426.4606) centre (-439.42, 430.86) ccw
  arc A202 (-398.78, 427.927) -> (-406.4, 432.3264) centre (-403.86, 427.927) ccw
  line L135 (-431.8, 417.6617) -> (-406.4, 432.3264)
  arc A203 (-431.8, 417.6617) -> (-431.8, 408.8629) centre (-429.26, 413.2623) ccw
  arc A204 (-462.28, 426.4606) -> (-454.66, 430.86) centre (-459.74, 430.86) ccw
  circle A205 centre (-449.58, 413.2623) radius 15.24 construction
  line L136 (-444.5, 430.86) -> (-444.5, 460.1894)
  arc A206 (-454.66, 460.1894) -> (-462.28, 464.5888) centre (-459.74, 460.1894) ccw
  line L137 (-454.66, 460.1894) -> (-454.66, 430.86)
  line L138 (-487.68, 449.9241) -> (-462.28, 464.5888)
  line L139 (-462.28, 426.4606) -> (-487.68, 441.1253)
  arc A207 (-487.68, 449.9241) -> (-487.68, 441.1253) centre (-485.14, 445.5247) ccw
  circle A208 centre (-393.7, 445.5247) radius 15.24 construction
  arc A209 (-375.92, 449.9241) -> (-375.92, 441.1253) centre (-373.38, 445.5247) ccw
  arc A210 (-388.62, 463.1223) -> (-381, 458.7229) centre (-383.54, 463.1223) ccw
  arc A211 (-350.52, 426.4606) -> (-342.9, 430.86) centre (-347.98, 430.86) ccw
  line L140 (-350.52, 426.4606) -> (-375.92, 441.1253)
  line L141 (-342.9, 460.1894) -> (-342.9, 430.86)
  line L142 (-375.92, 449.9241) -> (-350.52, 464.5888)
  line L143 (-355.6, 473.3876) -> (-381, 458.7229)
  arc A212 (-342.9, 460.1894) -> (-350.52, 464.5888) centre (-347.98, 460.1894) ccw
  arc A213 (-355.6, 473.3876) -> (-355.6, 482.1864) centre (-358.14, 477.787) ccw
  line L144 (-388.62, 463.1223) -> (-388.62, 492.4517)
  line L145 (-381, 496.8511) -> (-355.6, 482.1864)
  arc A214 (-350.52, 490.9852) -> (-342.9, 495.3846) centre (-347.98, 495.3846) ccw
  line L146 (-350.52, 490.9852) -> (-375.92, 505.6499)
  arc A215 (-375.92, 514.4487) -> (-375.92, 505.6499) centre (-373.38, 510.0493) ccw
  line L147 (-342.9, 524.714) -> (-342.9, 495.3846)
  line L148 (-375.92, 514.4487) -> (-350.52, 529.1134)
  line L149 (-355.6, 537.9123) -> (-381, 523.2476)
  arc A216 (-355.6, 537.9123) -> (-355.6, 546.7111) centre (-358.14, 542.3117) ccw
  line L150 (-381, 561.3758) -> (-355.6, 546.7111)
  arc A217 (-381, 561.3758) -> (-388.62, 556.9764) centre (-383.54, 556.9764) ccw
  line L151 (-388.62, 527.647) -> (-388.62, 556.9764)
  arc A218 (-431.8, 546.7111) -> (-431.8, 537.9123) centre (-429.26, 542.3117) ccw
  arc A219 (-436.88, 529.1134) -> (-444.5, 524.714) centre (-439.42, 524.714) ccw
  arc A220 (-406.4, 523.2476) -> (-398.78, 527.647) centre (-403.86, 527.647) ccw
  line L152 (-406.4, 523.2476) -> (-431.8, 537.9123)
  line L153 (-398.78, 556.9764) -> (-398.78, 527.647)
  line L154 (-431.8, 546.7111) -> (-406.4, 561.3758)
  arc A221 (-398.78, 556.9764) -> (-406.4, 561.3758) centre (-403.86, 556.9764) ccw
  line L155 (-436.88, 464.5888) -> (-411.48, 449.9241)
  line L156 (-398.78, 492.4517) -> (-398.78, 463.1223)
  arc A222 (-406.4, 458.7229) -> (-398.78, 463.1223) centre (-403.86, 463.1223) ccw
  line L157 (-406.4, 458.7229) -> (-431.8, 473.3876)
  line L158 (-421.64, 467.5217) -> (-426.72, 458.7229)
  arc A223 (-406.4, 458.7229) -> (-398.78, 463.1223) centre (-403.86, 463.1223) ccw
  arc A224 (-406.4, 458.7229) -> (-398.78, 463.1223) centre (-403.86, 463.1223) ccw
  line L159 (-406.4, 458.7229) -> (-431.8, 473.3876)
  line L160 (-406.4, 458.7229) -> (-431.8, 473.3876)
  line L161 (-398.78, 492.4517) -> (-398.78, 463.1223)
  line L162 (-398.78, 492.4517) -> (-398.78, 463.1223)
  line L163 (-431.8, 482.1864) -> (-406.4, 496.8511)
  line L164 (-411.48, 505.6499) -> (-436.88, 490.9852)
  line L165 (-411.48, 505.6499) -> (-436.88, 490.9852)
  line L166 (-431.8, 482.1864) -> (-406.4, 496.8511)
  line L167 (-431.8, 482.1864) -> (-406.4, 496.8511)
  arc A225 (-411.48, 505.6499) -> (-411.48, 514.4487) centre (-414.02, 510.0493) ccw
  arc A226 (-398.78, 492.4517) -> (-406.4, 496.8511) centre (-403.86, 492.4517) ccw
  arc A227 (-398.78, 492.4517) -> (-406.4, 496.8511) centre (-403.86, 492.4517) ccw
  line L168 (-398.78, 492.4517) -> (-398.78, 463.1223)
  arc A228 (-406.4, 458.7229) -> (-398.78, 463.1223) centre (-403.86, 463.1223) ccw
  arc A229 (-492.76, 561.3758) -> (-500.38, 556.9764) centre (-495.3, 556.9764) ccw
  arc A230 (-411.48, 441.1253) -> (-411.48, 449.9241) centre (-414.02, 445.5247) ccw
  line L169 (-431.8, 482.1864) -> (-406.4, 496.8511)
  line L170 (-406.4, 458.7229) -> (-431.8, 473.3876)
  arc A231 (-431.8, 482.1864) -> (-431.8, 473.3876) centre (-429.26, 477.787) ccw
  line L171 (-436.88, 464.5888) -> (-411.48, 449.9241)
  line L172 (-411.48, 441.1253) -> (-436.88, 426.4606)
  line L173 (-518.16, 394.1982) -> (-543.56, 408.8629)
  arc A232 (-543.56, 417.6617) -> (-543.56, 408.8629) centre (-541.02, 413.2623) ccw
  line L174 (-510.54, 427.927) -> (-510.54, 398.5976)
  line L175 (-543.56, 417.6617) -> (-518.16, 432.3264)
  arc A233 (-510.54, 427.927) -> (-518.16, 432.3264) centre (-515.62, 427.927) ccw
  line L176 (-523.24, 441.1253) -> (-548.64, 426.4606)
  arc A234 (-523.24, 441.1253) -> (-523.24, 449.9241) centre (-525.78, 445.5247) ccw
  line L177 (-556.26, 430.86) -> (-556.26, 460.1894)
  arc A235 (-556.26, 430.86) -> (-548.64, 426.4606) centre (-551.18, 430.86) ccw
  circle A236 centre (-505.46, 445.5247) radius 15.24 construction
  line L178 (-490.22, 445.5247) -> (-500.38, 445.5247)
  arc A237 (-487.68, 449.9241) -> (-487.68, 441.1253) centre (-485.14, 445.5247) ccw
  circle A238 centre (-505.46, 445.5247) radius 5.08
  line L179 (-518.16, 458.7229) -> (-543.56, 473.3876)
  arc A239 (-543.56, 482.1864) -> (-543.56, 473.3876) centre (-541.02, 477.787) ccw
  line L180 (-543.56, 482.1864) -> (-518.16, 496.8511)
  line L181 (-543.56, 482.1864) -> (-518.16, 496.8511)
  arc A240 (-518.16, 458.7229) -> (-510.54, 463.1223) centre (-515.62, 463.1223) ccw
  arc A241 (-518.16, 458.7229) -> (-510.54, 463.1223) centre (-515.62, 463.1223) ccw
  line L182 (-518.16, 458.7229) -> (-543.56, 473.3876)
  arc A242 (-548.64, 464.5888) -> (-556.26, 460.1894) centre (-551.18, 460.1894) ccw
  line L183 (-548.64, 464.5888) -> (-523.24, 449.9241)
  arc A243 (-492.76, 496.8511) -> (-500.38, 492.4517) centre (-495.3, 492.4517) ccw
  arc A244 (-518.16, 523.2476) -> (-510.54, 527.647) centre (-515.62, 527.647) ccw
  arc A245 (-510.54, 492.4517) -> (-518.16, 496.8511) centre (-515.62, 492.4517) ccw
  circle A246 centre (-505.46, 510.0493) radius 15.24 construction
  arc A247 (-487.68, 514.4487) -> (-487.68, 505.6499) centre (-485.14, 510.0493) ccw
  arc A248 (-492.76, 496.8511) -> (-500.38, 492.4517) centre (-495.3, 492.4517) ccw
  arc A249 (-500.38, 463.1223) -> (-492.76, 458.7229) centre (-495.3, 463.1223) ccw
  arc A250 (-500.38, 463.1223) -> (-492.76, 458.7229) centre (-495.3, 463.1223) ccw
  arc A251 (-500.38, 463.1223) -> (-492.76, 458.7229) centre (-495.3, 463.1223) ccw
  arc A252 (-518.16, 394.1982) -> (-510.54, 398.5976) centre (-515.62, 398.5976) ccw
  line L184 (-454.66, 460.1894) -> (-454.66, 430.86)
  arc A253 (-454.66, 460.1894) -> (-462.28, 464.5888) centre (-459.74, 460.1894) ccw
  arc A254 (-462.28, 426.4606) -> (-454.66, 430.86) centre (-459.74, 430.86) ccw
  arc A255 (-436.88, 464.5888) -> (-444.5, 460.1894) centre (-439.42, 460.1894) ccw
  line L185 (-444.5, 430.86) -> (-444.5, 460.1894)
  arc A256 (-444.5, 430.86) -> (-436.88, 426.4606) centre (-439.42, 430.86) ccw
  arc A257 (-467.36, 408.8629) -> (-467.36, 417.6617) centre (-469.9, 413.2623) ccw
  circle A258 centre (-449.58, 413.2623) radius 15.24 construction
  line L186 (-462.28, 426.4606) -> (-487.68, 441.1253)
  arc A259 (-492.76, 432.3264) -> (-500.38, 427.927) centre (-495.3, 427.927) ccw
  line L187 (-492.76, 432.3264) -> (-467.36, 417.6617)
  line L188 (-500.38, 398.5976) -> (-500.38, 427.927)
  line L189 (-467.36, 408.8629) -> (-492.76, 394.1982)
  arc A260 (-500.38, 398.5976) -> (-492.76, 394.1982) centre (-495.3, 398.5976) ccw
  circle A261 centre (-449.58, 477.787) radius 15.24 construction
  arc A262 (-444.5, 495.3846) -> (-436.88, 490.9852) centre (-439.42, 495.3846) ccw
  arc A263 (-462.28, 490.9852) -> (-454.66, 495.3846) centre (-459.74, 495.3846) ccw
  arc A264 (-411.48, 505.6499) -> (-411.48, 514.4487) centre (-414.02, 510.0493) ccw
  line L190 (-411.48, 505.6499) -> (-436.88, 490.9852)
  line L191 (-436.88, 529.1134) -> (-411.48, 514.4487)
  line L192 (-444.5, 495.3846) -> (-444.5, 524.714)
  line L193 (-454.66, 524.714) -> (-454.66, 495.3846)
  arc A265 (-436.88, 529.1134) -> (-444.5, 524.714) centre (-439.42, 524.714) ccw
  arc A266 (-454.66, 524.714) -> (-462.28, 529.1134) centre (-459.74, 524.714) ccw
  line L194 (-462.28, 490.9852) -> (-487.68, 505.6499)
  line L195 (-487.68, 514.4487) -> (-462.28, 529.1134)
  arc A267 (-467.36, 537.9123) -> (-467.36, 546.7111) centre (-469.9, 542.3117) ccw
  line L196 (-467.36, 537.9123) -> (-492.76, 523.2476)
  arc A268 (-500.38, 527.647) -> (-492.76, 523.2476) centre (-495.3, 527.647) ccw
  line L197 (-492.76, 561.3758) -> (-467.36, 546.7111)
  line L198 (-500.38, 527.647) -> (-500.38, 556.9764)
  line L199 (-510.54, 556.9764) -> (-510.54, 527.647)
  arc A269 (-510.54, 556.9764) -> (-518.16, 561.3758) centre (-515.62, 556.9764) ccw
  line L200 (-543.56, 546.7111) -> (-518.16, 561.3758)
  arc A270 (-543.56, 546.7111) -> (-543.56, 537.9123) centre (-541.02, 542.3117) ccw
  line L201 (-518.16, 523.2476) -> (-543.56, 537.9123)
  arc A271 (-556.26, 495.3846) -> (-548.64, 490.9852) centre (-551.18, 495.3846) ccw
  arc A272 (-543.56, 482.1864) -> (-543.56, 473.3876) centre (-541.02, 477.787) ccw
  arc A273 (-523.24, 505.6499) -> (-523.24, 514.4487) centre (-525.78, 510.0493) ccw
  line L202 (-523.24, 505.6499) -> (-548.64, 490.9852)
  line L203 (-548.64, 529.1134) -> (-523.24, 514.4487)
  line L204 (-556.26, 495.3846) -> (-556.26, 524.714)
  arc A274 (-548.64, 529.1134) -> (-556.26, 524.714) centre (-551.18, 524.714) ccw
  line L205 (-487.68, 449.9241) -> (-462.28, 464.5888)
  line L206 (-492.76, 496.8511) -> (-467.36, 482.1864)
  arc A275 (-467.36, 473.3876) -> (-467.36, 482.1864) centre (-469.9, 477.787) ccw
  line L207 (-467.36, 473.3876) -> (-492.76, 458.7229)
  line L208 (-482.6, 464.5888) -> (-477.52, 455.79)
  arc A276 (-467.36, 473.3876) -> (-467.36, 482.1864) centre (-469.9, 477.787) ccw
  arc A277 (-467.36, 473.3876) -> (-467.36, 482.1864) centre (-469.9, 477.787) ccw
  line L209 (-467.36, 473.3876) -> (-492.76, 458.7229)
  line L210 (-467.36, 473.3876) -> (-492.76, 458.7229)
  line L211 (-492.76, 496.8511) -> (-467.36, 482.1864)
  line L212 (-492.76, 496.8511) -> (-467.36, 482.1864)
  line L213 (-500.38, 463.1223) -> (-500.38, 492.4517)
  line L214 (-510.54, 492.4517) -> (-510.54, 463.1223)
  line L215 (-510.54, 492.4517) -> (-510.54, 463.1223)
  line L216 (-500.38, 463.1223) -> (-500.38, 492.4517)
  line L217 (-500.38, 463.1223) -> (-500.38, 492.4517)
  arc A278 (-510.54, 492.4517) -> (-518.16, 496.8511) centre (-515.62, 492.4517) ccw
  arc A279 (-492.76, 496.8511) -> (-500.38, 492.4517) centre (-495.3, 492.4517) ccw
  arc A280 (-492.76, 496.8511) -> (-500.38, 492.4517) centre (-495.3, 492.4517) ccw
  line L218 (-492.76, 496.8511) -> (-467.36, 482.1864)
  arc A281 (-467.36, 473.3876) -> (-467.36, 482.1864) centre (-469.9, 477.787) ccw
  arc A282 (-599.44, 449.9241) -> (-599.44, 441.1253) centre (-596.9, 445.5247) ccw
  arc A283 (-454.66, 460.1894) -> (-462.28, 464.5888) centre (-459.74, 460.1894) ccw
  line L219 (-500.38, 463.1223) -> (-500.38, 492.4517)
  line L220 (-467.36, 473.3876) -> (-492.76, 458.7229)
  arc A284 (-500.38, 463.1223) -> (-492.76, 458.7229) centre (-495.3, 463.1223) ccw
  line L221 (-487.68, 449.9241) -> (-462.28, 464.5888)
  line L222 (-454.66, 460.1894) -> (-454.66, 430.86)
  line L223 (-467.36, 344.3383) -> (-492.76, 329.6736)
  arc A285 (-500.38, 334.073) -> (-492.76, 329.6736) centre (-495.3, 334.073) ccw
  line L224 (-492.76, 367.8018) -> (-467.36, 353.1371)
  line L225 (-500.38, 334.073) -> (-500.38, 363.4024)
  arc A286 (-492.76, 367.8018) -> (-500.38, 363.4024) centre (-495.3, 363.4024) ccw
  line L226 (-510.54, 363.4024) -> (-510.54, 334.073)
  arc A287 (-510.54, 363.4024) -> (-518.16, 367.8018) centre (-515.62, 363.4024) ccw
  line L227 (-518.16, 329.6736) -> (-543.56, 344.3383)
  arc A288 (-518.16, 329.6736) -> (-510.54, 334.073) centre (-515.62, 334.073) ccw
  circle A289 centre (-505.46, 381) radius 15.24 construction
  line L228 (-497.84, 394.1982) -> (-502.92, 385.3994)
  arc A290 (-500.38, 398.5976) -> (-492.76, 394.1982) centre (-495.3, 398.5976) ccw
  circle A291 centre (-505.46, 381) radius 5.08
  line L229 (-523.24, 376.6006) -> (-548.64, 361.9359)
  arc A292 (-556.26, 366.3353) -> (-548.64, 361.9359) centre (-551.18, 366.3353) ccw
  line L230 (-556.26, 366.3353) -> (-556.26, 395.6647)
  line L231 (-556.26, 366.3353) -> (-556.26, 395.6647)
  arc A293 (-523.24, 376.6006) -> (-523.24, 385.3994) centre (-525.78, 381) ccw
  arc A294 (-523.24, 376.6006) -> (-523.24, 385.3994) centre (-525.78, 381) ccw
  line L232 (-523.24, 376.6006) -> (-548.64, 361.9359)
  arc A295 (-543.56, 353.1371) -> (-543.56, 344.3383) centre (-541.02, 348.7377) ccw
  line L233 (-543.56, 353.1371) -> (-518.16, 367.8018)
  arc A296 (-543.56, 417.6617) -> (-543.56, 408.8629) centre (-541.02, 413.2623) ccw
  arc A297 (-579.12, 408.8629) -> (-579.12, 417.6617) centre (-581.66, 413.2623) ccw
  arc A298 (-548.64, 400.0641) -> (-556.26, 395.6647) centre (-551.18, 395.6647) ccw
  circle A299 centre (-561.34, 413.2623) radius 15.24 construction
  arc A300 (-556.26, 430.86) -> (-548.64, 426.4606) centre (-551.18, 430.86) ccw
  arc A301 (-543.56, 417.6617) -> (-543.56, 408.8629) centre (-541.02, 413.2623) ccw
  arc A302 (-518.16, 394.1982) -> (-510.54, 398.5976) centre (-515.62, 398.5976) ccw
  arc A303 (-518.16, 394.1982) -> (-510.54, 398.5976) centre (-515.62, 398.5976) ccw
  arc A304 (-518.16, 394.1982) -> (-510.54, 398.5976) centre (-515.62, 398.5976) ccw
  arc A305 (-467.36, 344.3383) -> (-467.36, 353.1371) centre (-469.9, 348.7377) ccw
  line L234 (-492.76, 432.3264) -> (-467.36, 417.6617)
  arc A306 (-492.76, 432.3264) -> (-500.38, 427.927) centre (-495.3, 427.927) ccw
  arc A307 (-467.36, 408.8629) -> (-467.36, 417.6617) centre (-469.9, 413.2623) ccw
  arc A308 (-487.68, 449.9241) -> (-487.68, 441.1253) centre (-485.14, 445.5247) ccw
  line L235 (-462.28, 426.4606) -> (-487.68, 441.1253)
  arc A309 (-462.28, 426.4606) -> (-454.66, 430.86) centre (-459.74, 430.86) ccw
  arc A310 (-454.66, 395.6647) -> (-462.28, 400.0641) centre (-459.74, 395.6647) ccw
  circle A311 centre (-449.58, 413.2623) radius 15.24 construction
  line L236 (-467.36, 408.8629) -> (-492.76, 394.1982)
  arc A312 (-487.68, 385.3994) -> (-487.68, 376.6006) centre (-485.14, 381) ccw
  line L237 (-487.68, 385.3994) -> (-462.28, 400.0641)
  line L238 (-462.28, 361.9359) -> (-487.68, 376.6006)
  line L239 (-454.66, 395.6647) -> (-454.66, 366.3353)
  arc A313 (-462.28, 361.9359) -> (-454.66, 366.3353) centre (-459.74, 366.3353) ccw
  circle A314 centre (-505.46, 445.5247) radius 15.24 construction
  arc A315 (-518.16, 458.7229) -> (-510.54, 463.1223) centre (-515.62, 463.1223) ccw
  arc A316 (-523.24, 441.1253) -> (-523.24, 449.9241) centre (-525.78, 445.5247) ccw
  arc A317 (-510.54, 492.4517) -> (-518.16, 496.8511) centre (-515.62, 492.4517) ccw
  line L240 (-510.54, 492.4517) -> (-510.54, 463.1223)
  line L241 (-543.56, 482.1864) -> (-518.16, 496.8511)
  line L242 (-518.16, 458.7229) -> (-543.56, 473.3876)
  line L243 (-548.64, 464.5888) -> (-523.24, 449.9241)
  arc A318 (-543.56, 482.1864) -> (-543.56, 473.3876) centre (-541.02, 477.787) ccw
  arc A319 (-548.64, 464.5888) -> (-556.26, 460.1894) centre (-551.18, 460.1894) ccw
  line L244 (-523.24, 441.1253) -> (-548.64, 426.4606)
  line L245 (-556.26, 430.86) -> (-556.26, 460.1894)
  arc A320 (-566.42, 460.1894) -> (-574.04, 464.5888) centre (-571.5, 460.1894) ccw
  line L246 (-566.42, 460.1894) -> (-566.42, 430.86)
  arc A321 (-574.04, 426.4606) -> (-566.42, 430.86) centre (-571.5, 430.86) ccw
  line L247 (-599.44, 449.9241) -> (-574.04, 464.5888)
  line L248 (-574.04, 426.4606) -> (-599.44, 441.1253)
  line L249 (-604.52, 432.3264) -> (-579.12, 417.6617)
  arc A322 (-604.52, 432.3264) -> (-612.14, 427.927) centre (-607.06, 427.927) ccw
  line L250 (-612.14, 398.5976) -> (-612.14, 427.927)
  arc A323 (-612.14, 398.5976) -> (-604.52, 394.1982) centre (-607.06, 398.5976) ccw
  line L251 (-579.12, 408.8629) -> (-604.52, 394.1982)
  arc A324 (-574.04, 361.9359) -> (-566.42, 366.3353) centre (-571.5, 366.3353) ccw
  arc A325 (-556.26, 366.3353) -> (-548.64, 361.9359) centre (-551.18, 366.3353) ccw
  arc A326 (-566.42, 395.6647) -> (-574.04, 400.0641) centre (-571.5, 395.6647) ccw
  line L252 (-566.42, 395.6647) -> (-566.42, 366.3353)
  line L253 (-599.44, 385.3994) -> (-574.04, 400.0641)
  line L254 (-574.04, 361.9359) -> (-599.44, 376.6006)
  arc A327 (-599.44, 385.3994) -> (-599.44, 376.6006) centre (-596.9, 381) ccw
  line L255 (-500.38, 398.5976) -> (-500.38, 427.927)
  line L256 (-543.56, 417.6617) -> (-518.16, 432.3264)
  arc A328 (-510.54, 427.927) -> (-518.16, 432.3264) centre (-515.62, 427.927) ccw
  line L257 (-510.54, 427.927) -> (-510.54, 398.5976)
  line L258 (-510.54, 410.3294) -> (-500.38, 410.3294)
  arc A329 (-510.54, 427.927) -> (-518.16, 432.3264) centre (-515.62, 427.927) ccw
  arc A330 (-510.54, 427.927) -> (-518.16, 432.3264) centre (-515.62, 427.927) ccw
  line L259 (-510.54, 427.927) -> (-510.54, 398.5976)
  line L260 (-510.54, 427.927) -> (-510.54, 398.5976)
  line L261 (-543.56, 417.6617) -> (-518.16, 432.3264)
  line L262 (-543.56, 417.6617) -> (-518.16, 432.3264)
  line L263 (-518.16, 394.1982) -> (-543.56, 408.8629)
  line L264 (-548.64, 400.0641) -> (-523.24, 385.3994)
  line L265 (-548.64, 400.0641) -> (-523.24, 385.3994)
  line L266 (-518.16, 394.1982) -> (-543.56, 408.8629)
  line L267 (-518.16, 394.1982) -> (-543.56, 408.8629)
  arc A331 (-548.64, 400.0641) -> (-556.26, 395.6647) centre (-551.18, 395.6647) ccw
  arc A332 (-543.56, 417.6617) -> (-543.56, 408.8629) centre (-541.02, 413.2623) ccw
  arc A333 (-543.56, 417.6617) -> (-543.56, 408.8629) centre (-541.02, 413.2623) ccw
  line L268 (-543.56, 417.6617) -> (-518.16, 432.3264)
  arc A334 (-510.54, 427.927) -> (-518.16, 432.3264) centre (-515.62, 427.927) ccw
  arc A335 (-556.26, 301.8106) -> (-548.64, 297.4112) centre (-551.18, 301.8106) ccw
  arc A336 (-492.76, 432.3264) -> (-500.38, 427.927) centre (-495.3, 427.927) ccw
  line L269 (-518.16, 394.1982) -> (-543.56, 408.8629)
  line L270 (-510.54, 427.927) -> (-510.54, 398.5976)
  arc A337 (-518.16, 394.1982) -> (-510.54, 398.5976) centre (-515.62, 398.5976) ccw
  line L271 (-500.38, 398.5976) -> (-500.38, 427.927)
  line L272 (-492.76, 432.3264) -> (-467.36, 417.6617)
  line L273 (-398.78, 363.4024) -> (-398.78, 334.073)
  arc A338 (-406.4, 329.6736) -> (-398.78, 334.073) centre (-403.86, 334.073) ccw
  line L274 (-431.8, 353.1371) -> (-406.4, 367.8018)
  line L275 (-406.4, 329.6736) -> (-431.8, 344.3383)
  arc A339 (-431.8, 353.1371) -> (-431.8, 344.3383) centre (-429.26, 348.7377) ccw
  line L276 (-436.88, 335.5394) -> (-411.48, 320.8747)
  arc A340 (-436.88, 335.5394) -> (-444.5, 331.14) centre (-439.42, 331.14) ccw
  line L277 (-411.48, 312.0759) -> (-436.88, 297.4112)
  arc A341 (-411.48, 312.0759) -> (-411.48, 320.8747) centre (-414.02, 316.4753) ccw
  circle A342 centre (-449.58, 348.7377) radius 15.24 construction
  line L278 (-457.2, 361.9359) -> (-452.12, 353.1371)
  arc A343 (-462.28, 361.9359) -> (-454.66, 366.3353) centre (-459.74, 366.3353) ccw
  circle A344 centre (-449.58, 348.7377) radius 5.08
  line L279 (-454.66, 331.14) -> (-454.66, 301.8106)
  arc A345 (-462.28, 297.4112) -> (-454.66, 301.8106) centre (-459.74, 301.8106) ccw
  line L280 (-462.28, 297.4112) -> (-487.68, 312.0759)
  line L281 (-462.28, 297.4112) -> (-487.68, 312.0759)
  arc A346 (-454.66, 331.14) -> (-462.28, 335.5394) centre (-459.74, 331.14) ccw
  arc A347 (-454.66, 331.14) -> (-462.28, 335.5394) centre (-459.74, 331.14) ccw
  line L282 (-454.66, 331.14) -> (-454.66, 301.8106)
  arc A348 (-444.5, 301.8106) -> (-436.88, 297.4112) centre (-439.42, 301.8106) ccw
  line L283 (-444.5, 301.8106) -> (-444.5, 331.14)
  arc A349 (-500.38, 334.073) -> (-492.76, 329.6736) centre (-495.3, 334.073) ccw
  arc A350 (-510.54, 298.8777) -> (-518.16, 303.2771) centre (-515.62, 298.8777) ccw
  arc A351 (-487.68, 320.8747) -> (-487.68, 312.0759) centre (-485.14, 316.4753) ccw
  circle A352 centre (-505.46, 316.4753) radius 15.24 construction
  arc A353 (-518.16, 329.6736) -> (-510.54, 334.073) centre (-515.62, 334.073) ccw
  arc A354 (-500.38, 334.073) -> (-492.76, 329.6736) centre (-495.3, 334.073) ccw
  arc A355 (-467.36, 344.3383) -> (-467.36, 353.1371) centre (-469.9, 348.7377) ccw
  arc A356 (-467.36, 344.3383) -> (-467.36, 353.1371) centre (-469.9, 348.7377) ccw
  arc A357 (-467.36, 344.3383) -> (-467.36, 353.1371) centre (-469.9, 348.7377) ccw
  arc A358 (-398.78, 363.4024) -> (-406.4, 367.8018) centre (-403.86, 363.4024) ccw
  line L284 (-487.68, 385.3994) -> (-462.28, 400.0641)
  arc A359 (-487.68, 385.3994) -> (-487.68, 376.6006) centre (-485.14, 381) ccw
  arc A360 (-454.66, 395.6647) -> (-462.28, 400.0641) centre (-459.74, 395.6647) ccw
  arc A361 (-500.38, 398.5976) -> (-492.76, 394.1982) centre (-495.3, 398.5976) ccw
  line L285 (-467.36, 408.8629) -> (-492.76, 394.1982)
  arc A362 (-467.36, 408.8629) -> (-467.36, 417.6617) centre (-469.9, 413.2623) ccw